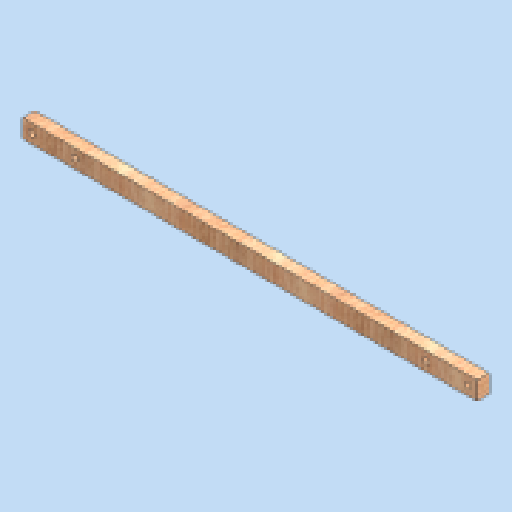
# Autodesk Inventor part: SeatBackSidePlate
Saved by Autodesk Inventor 2023 (Build 270158000, 158)
## iProperties
Created: 2026-03-22
Part Number: SeatBackSidePlate
Material: Wood (Birch)
Document SubType Name: Modeling
Designer: Nathann
Density: 0.55 g/cm^3
Appearance: Birch - Natural Polished
Author: Nathann
Autodesk Inventor part; units mm, degrees
ref_plane "YZ Plane" through (0, 0, 0) normal (1, 0, 0) x (0, 1, 0)
ref_plane "XZ Plane" through (0, 0, 0) normal (0, 1, 0) x (-1, 0, 0)
ref_plane "XY Plane" through (0, 0, 0) normal (0, 0, 1) x (1, 0, 0)
sketch "Sketch1" plane through (0, 0, 0) normal (0, 0, 1) x (1, 0, 0)
  line L0 (86.5042, -30) -> (-663.4958, -30)
  line L1 (-663.4958, -30) -> (-663.4958, 0)
  line L2 (-663.4958, 0) -> (86.5042, 0)
  line L3 (86.5042, 0) -> (86.5042, -30)
  circle A0 centre (71.5042, -15) radius 5
  circle A1 centre (1.5042, -15) radius 5
  circle A2 centre (-648.4958, -15) radius 5
  circle A3 centre (-578.4958, -15) radius 5.3247
  point P0 (0, 0)
  dimension "d0" = 30
  dimension "d1" = 750
  dimension "d2" = 10
  dimension "d3" = 15
  dimension "d4" = 15
  dimension "d5" = 15
  dimension "d6" = 10
  dimension "d7" = 70
  dimension "d8" = 15
  dimension "d9" = 10
  dimension "d10" = 15
  dimension "d11" = 15
  dimension "d12" = 70
  constraints: 8 end point, 4 centre point, 2 parallel, 1 horizontal, 1 perpendicular
  measures "d0" distance between parallel lines of L0 L2
  measures "d1" distance of L0.start L0.end
  measures "d2" diameter of A0
  measures "d3" distance from line of L3 A0.centre
  measures "d4" distance from line of L0 A0.centre
  measures "d5" distance from line of L0 A1.centre
  measures "d6" diameter of A1
  measures "d7" distance of A0.centre A1.centre
  measures "d8" distance from line of A2.centre L1
  measures "d9" diameter of A2
  measures "d10" distance from line of L0 A2.centre
  measures "d11" distance from line of L0 A3.centre
  measures "d12" distance of A2.centre A3.centre
extrude "Extrusion1" add sketch "Sketch1" along normal blind 20
body "Solid1"
